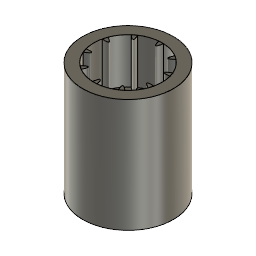
Untitled (Autodesk Fusion 360 design; units mm, degrees)
part number: 2026-02-11-18-54-11-585
Autodesk Fusion 360 part; units mm, degrees
sketch "Sketch1" plane through (0, 0, 0) normal (0, 0, 1) x (1, 0, 0)
  circle A0 centre (0, 0) radius 3.0101
  circle A1 centre (0, 0) radius 1.5
  spline S0 degree 5 poles (-0.2731, 2.9976) (-0.2642, 2.9604) (-0.2464, 2.8893) (-0.22, 2.7924) (-0.1852, 2.683) (-0.1426, 2.5818) (-0.101, 2.5193) (-0.0603, 2.4985) (-0.0207, 2.5212) (0.0179, 2.5857) (0.0555, 2.6889) (0.0849, 2.7997) (0.1067, 2.8978) (0.121, 2.9697) (0.1281, 3.0073) knots 0 0 0 0 0 0 0.1 0.2 0.3 0.4 0.5 0.6 0.7 0.8 0.9 1 1 1 1 1 1
  spline S1 degree 5 poles (0.1281, 3.0073) (0.1121, 3.0069) (0.08, 3.0062) (0.0318, 3.005) (-0.0324, 3.0035) (-0.1126, 3.0015) (-0.1768, 3) (-0.225, 2.9988) (-0.2571, 2.998) (-0.2731, 2.9976) knots 0 0 0 0 0 0 0.2 0.4 0.6 0.8 1 1 1 1 1 1
  spline S2 degree 5 poles (-1.9829, 2.2646) (-1.9538, 2.2398) (-1.8976, 2.1926) (-1.8193, 2.1298) (-1.7269, 2.0617) (-1.633, 2.0049) (-1.5625, 1.9788) (-1.5174, 1.9859) (-1.4987, 2.0275) (-1.5054, 2.1024) (-1.5356, 2.208) (-1.5769, 2.315) (-1.617, 2.4071) (-1.6477, 2.4737) (-1.664, 2.5083) knots 0 0 0 0 0 0 0.1 0.2 0.3 0.4 0.5 0.6 0.7 0.8 0.9 1 1 1 1 1 1
  spline S3 degree 5 poles (-1.664, 2.5083) (-1.6768, 2.4985) (-1.7023, 2.479) (-1.7406, 2.4498) (-1.7916, 2.4108) (-1.8554, 2.3621) (-1.9064, 2.3231) (-1.9447, 2.2938) (-1.9702, 2.2744) (-1.9829, 2.2646) knots 0 0 0 0 0 0 0.2 0.4 0.6 0.8 1 1 1 1 1 1
  spline S4 degree 5 poles (-2.9353, 0.6666) (-2.8972, 0.6636) (-2.824, 0.6585) (-2.7237, 0.6537) (-2.609, 0.6529) (-2.4996, 0.6622) (-2.4272, 0.6825) (-2.3949, 0.7147) (-2.4042, 0.7594) (-2.4537, 0.816) (-2.5401, 0.8837) (-2.6364, 0.946) (-2.723, 0.9969) (-2.787, 1.0328) (-2.8206, 1.0512) knots 0 0 0 0 0 0 0.1 0.2 0.3 0.4 0.5 0.6 0.7 0.8 0.9 1 1 1 1 1 1
  spline S5 degree 5 poles (-2.8206, 1.0512) (-2.8251, 1.0358) (-2.8343, 1.005) (-2.8481, 0.9589) (-2.8665, 0.8973) (-2.8894, 0.8204) (-2.9078, 0.7589) (-2.9216, 0.7127) (-2.9307, 0.6819) (-2.9353, 0.6666) knots 0 0 0 0 0 0 0.2 0.4 0.6 0.8 1 1 1 1 1 1
  spline S6 degree 5 poles (-2.7665, -1.1861) (-2.7339, -1.1661) (-2.6717, -1.1272) (-2.5877, -1.0721) (-2.4945, -1.0053) (-2.4114, -0.9335) (-2.3648, -0.8745) (-2.3576, -0.8295) (-2.3914, -0.7988) (-2.4647, -0.7821) (-2.5744, -0.7781) (-2.6889, -0.7844) (-2.7889, -0.794) (-2.8618, -0.8026) (-2.8997, -0.8075) knots 0 0 0 0 0 0 0.1 0.2 0.3 0.4 0.5 0.6 0.7 0.8 0.9 1 1 1 1 1 1
  spline S7 degree 5 poles (-2.8997, -0.8075) (-2.8944, -0.8226) (-2.8837, -0.8529) (-2.8678, -0.8983) (-2.8465, -0.9589) (-2.8198, -1.0346) (-2.7985, -1.0952) (-2.7825, -1.1406) (-2.7719, -1.1709) (-2.7665, -1.1861) knots 0 0 0 0 0 0 0.2 0.4 0.6 0.8 1 1 1 1 1 1
  spline S8 degree 5 poles (-1.541, -2.5857) (-1.5264, -2.5503) (-1.4989, -2.4823) (-1.4633, -2.3884) (-1.4272, -2.2795) (-1.4022, -2.1726) (-1.3991, -2.0975) (-1.4198, -2.0568) (-1.4652, -2.0519) (-1.5343, -2.0814) (-1.6254, -2.1427) (-1.7144, -2.2151) (-1.7896, -2.2817) (-1.8435, -2.3315) (-1.8713, -2.3577) knots 0 0 0 0 0 0 0.1 0.2 0.3 0.4 0.5 0.6 0.7 0.8 0.9 1 1 1 1 1 1
  spline S9 degree 5 poles (-1.8713, -2.3577) (-1.8581, -2.3668) (-1.8317, -2.385) (-1.792, -2.4124) (-1.7392, -2.4489) (-1.6731, -2.4945) (-1.6203, -2.531) (-1.5806, -2.5583) (-1.5542, -2.5766) (-1.541, -2.5857) knots 0 0 0 0 0 0 0.2 0.4 0.6 0.8 1 1 1 1 1 1
  spline S10 degree 5 poles (0.2731, -2.9976) (0.2642, -2.9604) (0.2464, -2.8893) (0.22, -2.7924) (0.1852, -2.683) (0.1426, -2.5818) (0.101, -2.5193) (0.0603, -2.4985) (0.0207, -2.5212) (-0.0179, -2.5857) (-0.0555, -2.6889) (-0.0849, -2.7997) (-0.1067, -2.8978) (-0.121, -2.9697) (-0.1281, -3.0073) knots 0 0 0 0 0 0 0.1 0.2 0.3 0.4 0.5 0.6 0.7 0.8 0.9 1 1 1 1 1 1
  spline S11 degree 5 poles (-0.1281, -3.0073) (-0.1121, -3.0069) (-0.08, -3.0062) (-0.0318, -3.005) (0.0324, -3.0035) (0.1126, -3.0015) (0.1768, -3) (0.225, -2.9988) (0.2571, -2.998) (0.2731, -2.9976) knots 0 0 0 0 0 0 0.2 0.4 0.6 0.8 1 1 1 1 1 1
  spline S12 degree 5 poles (1.9829, -2.2646) (1.9538, -2.2398) (1.8976, -2.1926) (1.8193, -2.1298) (1.7269, -2.0617) (1.633, -2.0049) (1.5625, -1.9788) (1.5174, -1.9859) (1.4987, -2.0275) (1.5054, -2.1024) (1.5356, -2.208) (1.5769, -2.315) (1.617, -2.4071) (1.6477, -2.4737) (1.664, -2.5083) knots 0 0 0 0 0 0 0.1 0.2 0.3 0.4 0.5 0.6 0.7 0.8 0.9 1 1 1 1 1 1
  spline S13 degree 5 poles (1.664, -2.5083) (1.6768, -2.4985) (1.7023, -2.479) (1.7406, -2.4498) (1.7916, -2.4108) (1.8554, -2.3621) (1.9064, -2.3231) (1.9447, -2.2938) (1.9702, -2.2744) (1.9829, -2.2646) knots 0 0 0 0 0 0 0.2 0.4 0.6 0.8 1 1 1 1 1 1
  spline S14 degree 5 poles (2.9353, -0.6666) (2.8972, -0.6636) (2.824, -0.6585) (2.7237, -0.6537) (2.609, -0.6529) (2.4996, -0.6622) (2.4272, -0.6825) (2.3949, -0.7147) (2.4042, -0.7594) (2.4537, -0.816) (2.5401, -0.8837) (2.6364, -0.946) (2.723, -0.9969) (2.787, -1.0328) (2.8206, -1.0512) knots 0 0 0 0 0 0 0.1 0.2 0.3 0.4 0.5 0.6 0.7 0.8 0.9 1 1 1 1 1 1
  spline S15 degree 5 poles (2.8206, -1.0512) (2.8251, -1.0358) (2.8343, -1.005) (2.8481, -0.9589) (2.8665, -0.8973) (2.8894, -0.8204) (2.9078, -0.7589) (2.9216, -0.7127) (2.9307, -0.6819) (2.9353, -0.6666) knots 0 0 0 0 0 0 0.2 0.4 0.6 0.8 1 1 1 1 1 1
  spline S16 degree 5 poles (2.7665, 1.1861) (2.7339, 1.1661) (2.6717, 1.1272) (2.5877, 1.0721) (2.4945, 1.0053) (2.4114, 0.9335) (2.3648, 0.8745) (2.3576, 0.8295) (2.3914, 0.7988) (2.4647, 0.7821) (2.5744, 0.7781) (2.6889, 0.7844) (2.7889, 0.794) (2.8618, 0.8026) (2.8997, 0.8075) knots 0 0 0 0 0 0 0.1 0.2 0.3 0.4 0.5 0.6 0.7 0.8 0.9 1 1 1 1 1 1
  spline S17 degree 5 poles (2.8997, 0.8075) (2.8944, 0.8226) (2.8837, 0.8529) (2.8678, 0.8983) (2.8465, 0.9589) (2.8198, 1.0346) (2.7985, 1.0952) (2.7825, 1.1406) (2.7719, 1.1709) (2.7665, 1.1861) knots 0 0 0 0 0 0 0.2 0.4 0.6 0.8 1 1 1 1 1 1
  spline S18 degree 5 poles (1.541, 2.5857) (1.5264, 2.5503) (1.4989, 2.4823) (1.4633, 2.3884) (1.4272, 2.2795) (1.4022, 2.1726) (1.3991, 2.0975) (1.4198, 2.0568) (1.4652, 2.0519) (1.5343, 2.0814) (1.6254, 2.1427) (1.7144, 2.2151) (1.7896, 2.2817) (1.8435, 2.3315) (1.8713, 2.3577) knots 0 0 0 0 0 0 0.1 0.2 0.3 0.4 0.5 0.6 0.7 0.8 0.9 1 1 1 1 1 1
  spline S19 degree 5 poles (1.8713, 2.3577) (1.8581, 2.3668) (1.8317, 2.385) (1.792, 2.4124) (1.7392, 2.4489) (1.6731, 2.4945) (1.6203, 2.531) (1.5806, 2.5583) (1.5542, 2.5766) (1.541, 2.5857) knots 0 0 0 0 0 0 0.2 0.4 0.6 0.8 1 1 1 1 1 1
  circle A2 centre (0, 0) radius 4
  point P0 (-0.0606, 2.5094)
  point P1 (-1.524, 1.9945)
  point P2 (-2.4053, 0.7178)
  point P3 (-2.3678, -0.8331)
  point P4 (-1.4259, -2.0657)
  point P5 (0.0606, -2.5094)
  point P6 (1.524, -1.9945)
  point P7 (2.4053, -0.7178)
  point P8 (2.3678, 0.8331)
  point P9 (1.4259, 2.0657)
  dimension "d2" = 360
  constraint coincident A0.centre A1.centre
  constraint concentric A0 A1
  constraint coincident A0 S0.start
  constraint coincident A0 S0.end
extrude "Extrude1" add sketch "Sketch1" along normal blind 8 contours S16 S17 | S14 S15 | S18 S19 | S12 S13 | S0 S1 | S10 S11 | S2 S3 | S8 S9 | S4 S5 | S6 S7 | A2 makes body 1 at (-2.6431, 0.9483, 4.7619)
extrude "Extrude2" add sketch "Sketch1" along normal blind 4 separate body contours A0 S0 S2 S4 S6 S8 S10 S12 S14 S16 S18 | A1 makes body 2
sketch "Sketch2" plane through (0, 0, 0) normal (0, 0, -1) x (1, 0, 0)
  arc A0 (-1.664, -2.5083) -> (-0.2731, -2.9976) centre (0, 0) ccw
  spline S0 degree 5 poles (-0.2731, -2.9976) (-0.2642, -2.9604) (-0.2464, -2.8893) (-0.22, -2.7924) (-0.1852, -2.683) (-0.1426, -2.5818) (-0.101, -2.5193) (-0.0603, -2.4985) (-0.0207, -2.5212) (0.0179, -2.5857) (0.0555, -2.6889) (0.0849, -2.7997) (0.1067, -2.8978) (0.121, -2.9697) (0.1281, -3.0073) knots 0 0 0 0 0 0 0.1 0.2 0.3 0.4 0.5 0.6 0.7 0.8 0.9 1 1 1 1 1 1
  arc A1 (0.1281, -3.0073) -> (1.541, -2.5857) centre (0, 0) ccw
  spline S1 degree 5 poles (1.541, -2.5857) (1.5264, -2.5503) (1.4989, -2.4823) (1.4633, -2.3884) (1.4272, -2.2795) (1.4022, -2.1726) (1.3991, -2.0975) (1.4198, -2.0568) (1.4652, -2.0519) (1.5343, -2.0814) (1.6254, -2.1427) (1.7144, -2.2151) (1.7896, -2.2817) (1.8435, -2.3315) (1.8713, -2.3577) knots 0 0 0 0 0 0 0.1 0.2 0.3 0.4 0.5 0.6 0.7 0.8 0.9 1 1 1 1 1 1
  arc A2 (1.8713, -2.3577) -> (2.7665, -1.1861) centre (0, 0) ccw
  spline S2 degree 5 poles (2.7665, -1.1861) (2.7339, -1.1661) (2.6717, -1.1272) (2.5877, -1.0721) (2.4945, -1.0053) (2.4114, -0.9335) (2.3648, -0.8745) (2.3576, -0.8295) (2.3914, -0.7988) (2.4647, -0.7821) (2.5744, -0.7781) (2.6889, -0.7844) (2.7889, -0.794) (2.8618, -0.8026) (2.8997, -0.8075) knots 0 0 0 0 0 0 0.1 0.2 0.3 0.4 0.5 0.6 0.7 0.8 0.9 1 1 1 1 1 1
  arc A3 (2.8997, -0.8075) -> (2.9353, 0.6666) centre (0, 0) ccw
  spline S3 degree 5 poles (2.9353, 0.6666) (2.8972, 0.6636) (2.824, 0.6585) (2.7237, 0.6537) (2.609, 0.6529) (2.4996, 0.6622) (2.4272, 0.6825) (2.3949, 0.7147) (2.4042, 0.7594) (2.4537, 0.816) (2.5401, 0.8837) (2.6364, 0.946) (2.723, 0.9969) (2.787, 1.0328) (2.8206, 1.0512) knots 0 0 0 0 0 0 0.1 0.2 0.3 0.4 0.5 0.6 0.7 0.8 0.9 1 1 1 1 1 1
  arc A4 (2.8206, 1.0512) -> (1.9829, 2.2646) centre (0, 0) ccw
  spline S4 degree 5 poles (1.9829, 2.2646) (1.9538, 2.2398) (1.8976, 2.1926) (1.8193, 2.1298) (1.7269, 2.0617) (1.633, 2.0049) (1.5625, 1.9788) (1.5174, 1.9859) (1.4987, 2.0275) (1.5054, 2.1024) (1.5356, 2.208) (1.5769, 2.315) (1.617, 2.4071) (1.6477, 2.4737) (1.664, 2.5083) knots 0 0 0 0 0 0 0.1 0.2 0.3 0.4 0.5 0.6 0.7 0.8 0.9 1 1 1 1 1 1
  arc A5 (1.664, 2.5083) -> (0.2731, 2.9976) centre (0, 0) ccw
  spline S5 degree 5 poles (0.2731, 2.9976) (0.2642, 2.9604) (0.2464, 2.8893) (0.22, 2.7924) (0.1852, 2.683) (0.1426, 2.5818) (0.101, 2.5193) (0.0603, 2.4985) (0.0207, 2.5212) (-0.0179, 2.5857) (-0.0555, 2.6889) (-0.0849, 2.7997) (-0.1067, 2.8978) (-0.121, 2.9697) (-0.1281, 3.0073) knots 0 0 0 0 0 0 0.1 0.2 0.3 0.4 0.5 0.6 0.7 0.8 0.9 1 1 1 1 1 1
  arc A6 (-0.1281, 3.0073) -> (-1.541, 2.5857) centre (0, 0) ccw
  spline S6 degree 5 poles (-1.541, 2.5857) (-1.5264, 2.5503) (-1.4989, 2.4823) (-1.4633, 2.3884) (-1.4272, 2.2795) (-1.4022, 2.1726) (-1.3991, 2.0975) (-1.4198, 2.0568) (-1.4652, 2.0519) (-1.5343, 2.0814) (-1.6254, 2.1427) (-1.7144, 2.2151) (-1.7896, 2.2817) (-1.8435, 2.3315) (-1.8713, 2.3577) knots 0 0 0 0 0 0 0.1 0.2 0.3 0.4 0.5 0.6 0.7 0.8 0.9 1 1 1 1 1 1
  arc A7 (-1.8713, 2.3577) -> (-2.7665, 1.1861) centre (0, 0) ccw
  spline S7 degree 5 poles (-2.7665, 1.1861) (-2.7339, 1.1661) (-2.6717, 1.1272) (-2.5877, 1.0721) (-2.4945, 1.0053) (-2.4114, 0.9335) (-2.3648, 0.8745) (-2.3576, 0.8295) (-2.3914, 0.7988) (-2.4647, 0.7821) (-2.5744, 0.7781) (-2.6889, 0.7844) (-2.7889, 0.794) (-2.8618, 0.8026) (-2.8997, 0.8075) knots 0 0 0 0 0 0 0.1 0.2 0.3 0.4 0.5 0.6 0.7 0.8 0.9 1 1 1 1 1 1
  arc A8 (-2.8997, 0.8075) -> (-2.9353, -0.6666) centre (0, 0) ccw
  spline S8 degree 5 poles (-2.9353, -0.6666) (-2.8972, -0.6636) (-2.824, -0.6585) (-2.7237, -0.6537) (-2.609, -0.6529) (-2.4996, -0.6622) (-2.4272, -0.6825) (-2.3949, -0.7147) (-2.4042, -0.7594) (-2.4537, -0.816) (-2.5401, -0.8837) (-2.6364, -0.946) (-2.723, -0.9969) (-2.787, -1.0328) (-2.8206, -1.0512) knots 0 0 0 0 0 0 0.1 0.2 0.3 0.4 0.5 0.6 0.7 0.8 0.9 1 1 1 1 1 1
  arc A9 (-2.8206, -1.0512) -> (-1.9829, -2.2646) centre (0, 0) ccw
  spline S9 degree 5 poles (-1.9829, -2.2646) (-1.9538, -2.2398) (-1.8976, -2.1926) (-1.8193, -2.1298) (-1.7269, -2.0617) (-1.633, -2.0049) (-1.5625, -1.9788) (-1.5174, -1.9859) (-1.4987, -2.0275) (-1.5054, -2.1024) (-1.5356, -2.208) (-1.5769, -2.315) (-1.617, -2.4071) (-1.6477, -2.4737) (-1.664, -2.5083) knots 0 0 0 0 0 0 0.1 0.2 0.3 0.4 0.5 0.6 0.7 0.8 0.9 1 1 1 1 1 1
  circle A10 centre (0, 0) radius 3.0101
  constraint concentric A0 A10
extrude "Extrude3" cut sketch "Sketch2" against normal blind 3 bodies 1 2
extrude "Extrude4" add 1 faces at (3.6547, -0.2264, 0) along direction (0, 0, -1) blind 2 on bodies 1 bodies 1
